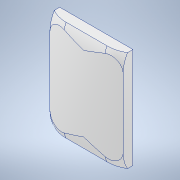
# Autodesk Inventor part: kühlblock
Saved by Autodesk Inventor 2021 (Build 250183000, 183)
## iProperties
Created: 2021-07-14
Part Number: kühlblock
Material: Aluminium 6061
Document SubType Name: Modeling
Designer: Simon
Density: 2.7 g/cm^3
Appearance: Aluminium - flach
Author: Simon
Autodesk Inventor part; units mm, degrees
ref_plane "YZ Plane" through (0, 0, 0) normal (1, 0, 0) x (0, 1, 0)
ref_plane "XZ Plane" through (0, 0, 0) normal (0, 1, 0) x (-1, 0, 0)
ref_plane "XY Plane" through (0, 0, 0) normal (0, 0, 1) x (1, 0, 0)
sketch "Skizze1" plane through (0, 0, 0) normal (0, 0, 1) x (1, 0, 0)
  line L0 (-43, 59) -> (43, 59)
  line L1 (43, 59) -> (43, -59)
  line L2 (43, -59) -> (-43, -59)
  line L3 (-43, -59) -> (-43, 59)
  point P0 (0, 0)
  point P1 (0, 59)
  point P2 (-43, 0)
  dimension "d0" = 86
  dimension "d1" = 118
  constraints: 8 end point, 2 midpoint, 2 parallel, 1 horizontal, 1 horizontal alignment, 1 perpendicular, 1 vertical alignment
  measures "d0" distance between parallel lines of L3 L1
  measures "d1" distance between parallel lines of L2 L0
extrude "Extrusion1" add sketch "Skizze1" against normal blind 14.9
sketch "Skizze2" plane through (0, 0, -14.9) normal (0, 0, -1) x (-1, 0, 0)
  line L0 (-43, -59) -> (43, -59) projected
  point P0 (0, 0)
  point P1 (-24, 0)
  point P2 (24, 0)
  point P3 (24, -36)
  point P4 (-24, -36)
  dimension "d4" = 36
  dimension "d5" = 48
  dimension "d6" = 23
  dimension "d7" = 24
  constraints: 2 horizontal alignment, 2 vertical alignment
  measures "d4" distance of point (24, -36) point (24, 0)
  measures "d5" distance of point (-24, 0) point (24, 0)
  measures "d6" distance from line of L0 point (-24, -36)
  measures "d7" distance of point (0, 0) point (-24, 0)
hole "Bohrung1" at (24, 0, -14.9) at (-24, 0, -14.9) at (-24, -36, -14.9) at (24, -36, -14.9) direction (0, 0, 1) diameter 3.242 depth 11.8 tip angle 118
sketch "Skizze3" plane through (0, 0, 0) normal (0, 0, 1) x (1, 0, 0)
  line L0 (-24, 44) -> (24, 44)
  line L1 (28, 40) -> (28, -40)
  line L2 (24, -44) -> (-24, -44)
  line L3 (-28, -40) -> (-28, 40)
  arc A0 (-28, -40) -> (-24, -44) centre (-24, -40) ccw
  arc A1 (-24, 44) -> (-28, 40) centre (-24, 40) ccw
  arc A2 (28, 40) -> (24, 44) centre (24, 40) ccw
  arc A3 (24, -44) -> (28, -40) centre (24, -40) ccw
  line L4 (43, -59) -> (43, 59) projected
  line L5 (-43, 59) -> (-43, -59) projected
  line L6 (43, 59) -> (-43, 59) projected
  line L7 (-43, -59) -> (43, -59) projected
  point P0 (0, 0)
  dimension "d15" = 4
  dimension "d16" = 15
  dimension "d17" = 15
  dimension "d18" = 15
  dimension "d19" = 15
  constraints: 8 end point, 8 point on circle, 8 tangent, 4 centre point, 3 equal radius, 2 parallel, 1 horizontal, 1 perpendicular
  measures "d15" radius of A2
  measures "d16" distance between parallel lines of L4 L1
  measures "d17" distance between parallel lines of L5 L3
  measures "d18" distance between parallel lines of L6 L0
  measures "d19" distance between parallel lines of L7 L2
sketch "Skizze4" plane through (0, 0, 0) normal (1, 0, 0) x (0, 1, 0)
  arc A0 (-44, 0) -> (-67, -8.688) centre (-44, -34.7882) ccw
  line L0 (59, 0) -> (-59, 0) projected
  line L1 (-44, 0) -> (-67, 0)
  line L2 (-67, 0) -> (-67, -8.688)
  line L3 (-59, 0) -> (-59, -14.9) projected
  line L4 (59, -14.9) -> (-59, -14.9) projected
  point P0 (0, 0)
  point P1 (-59, -3.4)
  dimension "d20" = 23
  dimension "d21" = 11.5
  constraints: 4 end point, 3 point on circle, 2 point on line, 1 centre point, 1 perpendicular, 1 tangent
  measures "d20" distance from line of point (-44, 0) L2
  measures "d21" distance from line of L4 point (-59, -3.4)
sweep "Sweeping1" cut profiles "Skizze4" path "Skizze3" path curves L2 A3 L1 A2 L0 A1 L3 A0
sketch "Skizze5" plane through (0, 0, 0) normal (0, 1, 0) x (-1, 0, 0)
  line L0 (24, 0) -> (-24, 0) projected
  line L1 (-43, -3.4) -> (-43, -8.5741) projected
  line L2 (-43, -8.5741) -> (-43, -14.9) projected
  line L3 (-43, -8.5741) -> (-43, -14.9) projected
  line L4 (-43, -8.5741) -> (-43, -3.4) projected
  line L5 (43, -8.5741) -> (43, -3.4) projected
  line L6 (43, -3.4) -> (43, -8.5741) projected
  line L7 (43, -8.5741) -> (43, -14.9) projected
  line L8 (43, -8.5741) -> (43, -14.9) projected
  arc A0 (43, -3.4) -> (-43, -3.4) centre (0, -273.6118) ccw
  line L9 (43, -3.4) -> (43, 1)
  line L10 (43, 1) -> (-43, 1)
  line L11 (-43, 1) -> (-43, -3.4)
  point P0 (0, 0)
  point P1 (43, -5.987)
  point P2 (-43, -5.987)
  dimension "d24" = 1
  constraints: 6 end point, 2 midpoint, 2 perpendicular, 2 point on circle, 2 point on line, 1 centre point, 1 horizontal alignment, 1 tangent, 1 vertical
  measures "d24" distance between parallel lines of L10 L0
extrude "Extrusion2" cut sketch "Skizze5" along normal through all both and the other way through all
equation "\"d7\" = 0.5 * d5"
equation "\"d17\" = d16"
